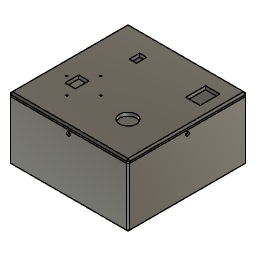
Omega (Autodesk Fusion 360 design; units mm, degrees)
Autodesk Fusion 360 part; units mm, degrees
sketch "Sketch1" plane through (0, 0, 0) normal (0, 0, 1) x (1, 0, 0) in component "Base"
  line L0 (875, 875) -> (-875, 875)
  line L1 (-875, 875) -> (-875, -875)
  line L2 (-875, -875) -> (875, -875)
  line L3 (875, -875) -> (875, 875)
  line L4 (875, 875) -> (-875, -875) construction
  line L5 (-875, 875) -> (875, -875) construction
  dimension "d1" = 1750
  dimension "d2" = 1750
  constraint horizontal L0
  constraint perpendicular L0 L1
  constraint parallel L0 L2
  constraint parallel L1 L3
  constraint coincident L4 origin
  constraint coincident L5 origin
  measures "d1" distance of L1.end L2.end
  measures "d2" distance of L0.end L1.end
  measures "d23" diameter of origin
extrude "Extrude1" add sketch "Sketch1" along normal blind 875 makes body 1 in component "Base"
sketch "Sketch2" plane through (0, 0, 875) normal (0, 0, 1) x (-1, 0, 0) in component "Base"
  line L0 (-875, 875) -> (-875, -875)
  line L1 (-875, -875) -> (875, -875)
  line L2 (875, -875) -> (875, 875)
  line L3 (875, 875) -> (-875, 875)
  line L4 (833, 833) -> (-833, 833)
  line L5 (-833, 833) -> (-833, -833)
  line L6 (-833, -833) -> (833, -833)
  line L7 (833, -833) -> (833, 833)
  dimension "d5" = -42
extrude "Extrude2" cut sketch "Sketch2" against normal blind 850 contours L4 L5 L6 L7 bodies 1 in component "Base"
sketch "Sketch1 (2)" plane through (0, 0, 875) normal (0, 0, 1) x (-1, 0, 0) in component "Top"
  line L0 (-833, 833) -> (833, 833)
  line L1 (833, 833) -> (833, -833)
  line L2 (833, -833) -> (-833, -833)
  line L3 (-833, -833) -> (-833, 833)
  line L4 (875, 875) -> (-875, 875)
  line L5 (-875, 875) -> (-875, -875)
  line L6 (-875, -875) -> (875, -875)
  line L7 (875, -875) -> (875, 875)
sketch "Sketch2 (2)" plane through (0, 0, 875) normal (0, 0, 1) x (-1, 0, 0) in component "Top"
sketch "Sketch3" plane through (0, 0, 875) normal (0, 0, 1) x (-1, 0, 0) in component "Top"
sketch "Sketch4" plane through (0, 0, 875) normal (0, 0, 1) x (-1, 0, 0) in component "Top"
  line L0 (-875, -875) -> (875, -875)
  line L1 (-875, 875) -> (-875, -875)
  line L2 (875, 875) -> (-875, 875)
  line L3 (875, -875) -> (875, 875)
  line L4 (-405, -425) -> (405, -425)
  line L5 (405, -425) -> (405, -575)
  line L6 (405, -575) -> (-405, -575)
  line L7 (-405, -575) -> (-405, -425)
  line L8 (-405, -425) -> (405, -575) construction
  line L9 (405, -425) -> (-405, -575) construction
  line L10 (300.7264, -425) -> (400.7264, -425)
  line L11 (400.7264, -425) -> (400.7264, -575)
  line L12 (400.7264, -575) -> (300.7264, -575)
  line L13 (300.7264, -575) -> (300.7264, -425)
  line L14 (300.7264, -425) -> (400.7264, -575) construction
  line L15 (400.7264, -425) -> (300.7264, -575) construction
  line L16 (425, 350) -> (575, 350)
  line L17 (575, 350) -> (575, 150)
  line L18 (575, 150) -> (425, 150)
  line L19 (425, 150) -> (425, 350)
  line L20 (425, 350) -> (575, 150) construction
  line L21 (575, 350) -> (425, 150) construction
  circle A0 centre (-350, 350) radius 125
  circle A1 centre (400, 0) radius 12.5
  circle A2 centre (400, 500) radius 12.5
  circle A3 centre (150, 250) radius 12.5
  circle A4 centre (650, 250) radius 12.5
  line L22 (-705, -355) -> (-495, -355)
  line L23 (-495, -355) -> (-495, -645)
  line L24 (-495, -645) -> (-705, -645)
  line L25 (-705, -645) -> (-705, -355)
  line L26 (-705, -355) -> (-495, -645) construction
  line L27 (-495, -355) -> (-705, -645) construction
  line L28 (230, 380) -> (570, 380)
  line L29 (570, 380) -> (570, 120)
  line L30 (570, 120) -> (230, 120)
  line L31 (230, 120) -> (230, 380)
  line L32 (230, 380) -> (570, 120) construction
  line L33 (570, 380) -> (230, 120) construction
  point P0 (0, -500)
  point P1 (350.7264, -500)
  point P2 (500, 250)
  point P3 (-600, -500)
  point P4 (400, 250)
  dimension "d14" = 810
  dimension "d15" = 150
  dimension "d16" = 100
  dimension "d17" = 150
  dimension "d18" = 150
  dimension "d19" = 200
  dimension "d20" = 250
  dimension "d21" = 25
  dimension "d22" = 25
  dimension "d23" = 25
  dimension "d24" = 25
  dimension "d25" = 210
  dimension "d26" = 290
  dimension "d27" = 340
  dimension "d28" = 260
  constraint horizontal L4
  constraint perpendicular L4 L5
  constraint parallel L4 L6
  constraint parallel L5 L7
  constraint coincident L8 P0
  constraint coincident L9 P0
  constraint horizontal L10
  constraint perpendicular L10 L11
  constraint parallel L10 L12
  constraint parallel L11 L13
  constraint coincident L14 P1
  constraint coincident L15 P1
  constraint horizontal L16
  constraint perpendicular L16 L17
  constraint parallel L16 L18
  constraint parallel L17 L19
  constraint coincident L20 P2
  constraint coincident L21 P2
  constraint horizontal L22
  constraint perpendicular L22 L23
  constraint parallel L22 L24
  constraint parallel L23 L25
  constraint coincident L26 P3
  constraint coincident L27 P3
  constraint horizontal L28
  constraint perpendicular L28 L29
  constraint parallel L28 L30
  constraint parallel L29 L31
  constraint coincident L32 P4
  constraint coincident L33 P4
  measures "d14" distance of L5.end L6.end
  measures "d15" distance of L4.end L5.end
  measures "d16" distance of L11.end L12.end
  measures "d17" distance of L10.end L11.end
  measures "d18" distance of L17.end L18.end
  measures "d19" distance of L16.end L17.end
  measures "d20" diameter of A0
  measures "d21" diameter of A1
  measures "d22" diameter of A2
  measures "d23" diameter of A3
  measures "d24" diameter of A4
  measures "d25" distance of L23.end L24.end
  measures "d26" distance of L22.end L23.end
  measures "d27" distance of L29.end L30.end
  measures "d28" distance of L28.end L29.end
extrude "Extrude1'" add sketch "Sketch1 (2)" sketch "Sketch4" along normal blind 50 separate body of sketch 2 contours L0 L1 L2 L3 | L4 L6 L7 L13 | L16 L18 L19 L28 L29 L30 L31 makes body 2 in component "Top"
sketch "Sketch1 (3)" plane through (0, 0, 875) normal (0, 0, 1) x (-1, 0, 0)
  line L0 (425, 150) -> (575, 150)
  line L1 (575, 150) -> (575, 350)
  line L2 (575, 350) -> (425, 350)
  line L3 (425, 350) -> (425, 150)
  line L4 (300.7264, -575) -> (405, -575)
  line L5 (405, -575) -> (405, -425)
  line L6 (405, -425) -> (300.7264, -425)
  line L7 (300.7264, -425) -> (300.7264, -575)
  line L8 (-705, -645) -> (-495, -645)
  line L9 (-495, -645) -> (-495, -355)
  line L10 (-495, -355) -> (-705, -355)
  line L11 (-705, -355) -> (-705, -645)
  circle A0 centre (650, 250) radius 12.5
  circle A1 centre (150, 250) radius 12.5
  circle A2 centre (400, 500) radius 12.5
  circle A3 centre (400, 0) radius 12.5
  circle A4 centre (-350, 350) radius 125
  line L12 (875, 875) -> (875, -875)
  line L13 (875, -875) -> (-875, -875)
  line L14 (-875, -875) -> (-875, 875)
  line L15 (-875, 875) -> (875, 875)
  line L16 (-825, 825) -> (825, 825)
  line L17 (825, 825) -> (825, -825)
  line L18 (825, -825) -> (-825, -825)
  line L19 (-825, -825) -> (-825, 825)
  line L20 (-775, 775) -> (775, 775)
  line L21 (775, 775) -> (775, -775)
  line L22 (775, -775) -> (-775, -775)
  line L23 (-775, -775) -> (-775, 775)
  dimension "d31" = 50
  dimension "d32" = 100
extrude "Extrude2'" add sketch "Sketch1 (3)" against normal blind 100 contours L16 L17 L18 L19 bodies 2 in component "Top"
sketch "Sketch2 (3)" plane through (0, -775, 0) normal (0, 1, 0) x (-1, 0, 0)
  line L0 (775, 875) -> (-775, 875)
  line L1 (-775, 875) -> (-775, 775)
  line L2 (-775, 775) -> (775, 775)
  line L3 (775, 775) -> (775, 875)
  line L4 (0, 875) -> (0, 775) construction
  line L5 (15.7328, 797.75) -> (31.4656, 825)
  line L6 (31.4656, 825) -> (15.7328, 852.25)
  line L7 (15.7328, 852.25) -> (-15.7328, 852.25)
  line L8 (-15.7328, 852.25) -> (-31.4656, 825)
  line L9 (-31.4656, 825) -> (-15.7328, 797.75)
  line L10 (-15.7328, 797.75) -> (15.7328, 797.75)
  circle A0 centre (0, 825) radius 19
  point P0 (0, 825)
  dimension "d35" = 27.25
  dimension "d36" = 38
  constraint midpoint L0 L4.start
  constraint midpoint L2 L4.end
  constraint midpoint L4 P0
  constraint coincident P0 A0.centre
  measures "d35" distance of P0 L10
  measures "d36" diameter of A0
extrude "Extrude3" cut sketch "Sketch2 (3)" against normal blind 232.934 contours A0 bodies 1 in component "Base"
extrude "Extrude3'" cut sketch "Sketch2 (3)" against normal blind 232.934 contours A0 bodies 2 in component "Top"
extrude "Extrude4" cut sketch "Sketch2 (3)" against normal blind 25 contours L5 L6 L7 L8 L9 L10 bodies 2 in component "Top"
sketch "Sketch3 (2)" plane through (0, -875, 0) normal (0, -1, 0) x (1, 0, 0)
  circle A0 centre (0, 825) radius 19
  line L0 (-875, 0) -> (875, 0)
  line L1 (875, 0) -> (875, 875)
  line L2 (875, 875) -> (-875, 875)
  line L3 (-875, 875) -> (-875, 0)
  circle A1 centre (0, 825) radius 27.5
  dimension "d53" = 55
  constraint concentric A0 A1
  measures "d53" diameter of A1
extrude "Extrude4'" cut sketch "Sketch3 (2)" against normal blind 25 contours A1 bodies 1 in component "Base"
pattern_circular "C-Pattern1" count 4 over 360 about axis through (0, 0, 1.75) along (0, 0, 1) of "Extrude3", "Extrude4'" in component "Base"
pattern_circular "C-Pattern1'" count 4 over 360 about axis through (0, 0, 1.75) along (0, 0, 1) of "Extrude3'", "Extrude4" in component "Top"
chamfer "Chamfer1" distance 25 angle 45 8 edges at (875, 0, 0) (875, -875, 437.5) (0, -875, 0) (875, 875, 437.5) (0, 875, 0) (-875, 875, 437.5) (-875, 0, 0) (-875, -875, 437.5) on bodies 1 in component "Base"
chamfer "Chamfer1'" distance 25 angle 45 8 edges at (-875, -875, 900) (-875, 0, 925) (0, -875, 925) (0, 875, 925) (875, 0, 925) (875, 875, 900) (875, -875, 900) (-875, 875, 900) on bodies 2 in component "Top"
scale "Scale1" factor 0.1 about (0, 0, 0) bodies 2 in component "Top"
scale "Scale1'" factor 0.1 about (0, 0, 0) bodies 1 in component "Base"
move_face "OffsetFaces1" offset -0.2 4 faces at (55.6311, -82.5, 82.5537) (82.5, 55.6311, 82.5537) (-82.5, -55.6311, 82.5537) (-55.6311, 82.5, 82.5537) on bodies 2 in component "Top"
chamfer "Chamfer2" distance 2.5 angle 45 8 edges at (82.3, -82.3, 82.5) (82.3, 82.3, 82.5) (-82.3, 82.3, 82.5) (-77.5, 77.5, 82.5) (-77.5, -77.5, 82.5) (-82.3, -82.3, 82.5) (77.5, -77.5, 82.5) (77.5, 77.5, 82.5) on bodies 2 in component "Top"
component "Base" placed x (1, 0, 0) y (0, 1, 0) z (0, 0, 1) at (0, 0, 0)
component "Top" placed x (1, 0, 0) y (0, 1, 0) z (0, 0, 1) at (0, 0, 0)
equation "d32 = 50 mm + 50 mm"
equation "d35 = ( 54.5 / 2 ) * 1 mm"
